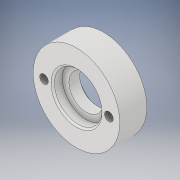
# Autodesk Inventor part: Корпус
Saved by Autodesk Inventor 2019.3 (Build 233278000, 278)
## iProperties
Created: 2020-04-01
Part Number: Корпус
Material: Типовые
Document SubType Name: Modeling
Designer: Admin
Density: 1 g/cm^3
Appearance: По умолчанию
Mass: 91.629 g
Surface Area: 184.335 cm^2
Volume: 91.629 cm^3
Author: Admin
Autodesk Inventor part; units mm, degrees
ref_plane "YZ Plane" through (0, 0, 0) normal (1, 0, 0) x (0, 1, 0)
ref_plane "XZ Plane" through (0, 0, 0) normal (0, 1, 0) x (-1, 0, 0)
ref_plane "XY Plane" through (0, 0, 0) normal (0, 0, 1) x (1, 0, 0)
sketch "Эскиз1" plane through (0, 0, 0) normal (0, 0, 1) x (1, 0, 0)
  circle A0 centre (0, 0) radius 40
  dimension "d0" = 80
  constraints: 1 centre point, 1 coincident
  measures "d0" diameter of A0
extrude "Выдавливание1" add sketch "Эскиз1" along normal blind 25
sketch "Эскиз2" plane through (0, 0, 25) normal (0, 0, 1) x (1, 0, 0)
  circle A0 centre (0, 0) radius 22
  dimension "d3" = 44
  constraints: 1 centre point, 1 coincident
  measures "d3" diameter of A0
extrude "Выдавливание2" cut sketch "Эскиз2" against normal blind 9
sketch "Эскиз3" plane through (0, 0, 0) normal (0, 0, -1) x (-1, 0, 0)
  circle A0 centre (0, 0) radius 24
  dimension "d6" = 48
  constraints: 1 centre point, 1 coincident
  measures "d6" diameter of A0
extrude "Выдавливание3" cut sketch "Эскиз3" against normal blind 6
sketch "Эскиз4" plane through (0, 0, 6) normal (0, 0, -1) x (-1, 0, 0)
  circle A0 centre (0, 0) radius 16
  dimension "d9" = 32
  constraints: 1 centre point, 1 coincident
  measures "d9" diameter of A0
extrude "Выдавливание4" cut sketch "Эскиз4" against normal through all
chamfer "Фаска1" distance 1.6 angle 45 1 edges at (-22, 0, 25)
sketch "Эскиз5" plane through (0, 0, 25) normal (0, 0, 1) x (1, 0, 0)
  point P0 (0, 0)
  point P1 (-30, 0)
  point P2 (30, 0)
  dimension "d15" = 60
  dimension "d16" = 30
  measures "d15" distance of point (30, 0) point (-30, 0)
  measures "d16" distance of point (-30, 0) point (0, 0)
hole "Отверстие2" at (-30, 0, 25) at (30, 0, 25) direction (0, 0, -1) diameter 8 depth 16.75 tip angle 120
thread "Резьба1" size "M8x1.25" class "6H" standard "ANSI Metric M Profile" length 10.5
thread "Резьба2" size "M8x1.25" class "6H" standard "ANSI Metric M Profile" length 10.5
